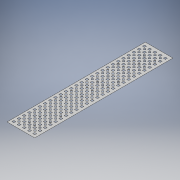
# Autodesk Inventor part: 5sqr metal plate
Saved by Autodesk Inventor 2018 (Build 220112000, 112)
## iProperties
Created: 2018-11-08
Part Number: 5sqr metal plate
Material: Generic
Document SubType Name: Modeling
Designer: USER
Density: 1 g/cm^3
Appearance: Default
Author: USER
Autodesk Inventor part; units mm, degrees
(part 1 of 2)
ref_plane "YZ Plane" through (0, 0, 0) normal (1, 0, 0) x (0, 1, 0)
ref_plane "XZ Plane" through (0, 0, 0) normal (0, 1, 0) x (-1, 0, 0)
ref_plane "XY Plane" through (0, 0, 0) normal (0, 0, 1) x (1, 0, 0)
sketch "Sketch1" plane through (0, 0, 0) normal (0, 1, 0) x (-1, 0, 0)
  line L0 (0, 0) -> (63, 0)
  line L1 (63, 0) -> (63, -315)
  line L2 (63, -315) -> (0, -315)
  line L3 (0, -315) -> (0, 0)
  dimension "d0" = 63
  dimension "d1" = 315
  constraints: 8 end point, 2 parallel, 1 horizontal, 1 perpendicular
  measures "d0" distance of L1.end L2.end
  measures "d1" distance of L0.end L1.end
extrude "Extrusion1" add sketch "Sketch1" along normal blind 0.1
sketch "Sketch2" plane through (0, 0.1, 0) normal (0, 1, 0) x (1, 0, 0)
  line L0 (-58.2087, 6.1745) -> (-53.6367, 6.1745)
  line L1 (-53.6367, 6.1745) -> (-53.6367, 10.7465)
  line L2 (-53.6367, 10.7465) -> (-58.2087, 10.7465)
  line L3 (-58.2087, 10.7465) -> (-58.2087, 6.1745)
  line L4 (-58.2087, 22.6465) -> (-58.2087, 18.0745)
  line L5 (-58.2087, 18.0745) -> (-53.6367, 18.0745)
  line L6 (-53.6367, 18.0745) -> (-53.6367, 22.6465)
  line L7 (-53.6367, 22.6465) -> (-58.2087, 22.6465)
  line L8 (-58.2087, 34.5465) -> (-58.2087, 29.9745)
  line L9 (-58.2087, 29.9745) -> (-53.6367, 29.9745)
  line L10 (-53.6367, 29.9745) -> (-53.6367, 34.5465)
  line L11 (-53.6367, 34.5465) -> (-58.2087, 34.5465)
  line L12 (-58.2087, 46.4465) -> (-58.2087, 41.8745)
  line L13 (-58.2087, 41.8745) -> (-53.6367, 41.8745)
  line L14 (-53.6367, 41.8745) -> (-53.6367, 46.4465)
  line L15 (-53.6367, 46.4465) -> (-58.2087, 46.4465)
  line L16 (-58.2087, 58.3465) -> (-58.2087, 53.7745)
  line L17 (-58.2087, 53.7745) -> (-53.6367, 53.7745)
  line L18 (-53.6367, 53.7745) -> (-53.6367, 58.3465)
  line L19 (-53.6367, 58.3465) -> (-58.2087, 58.3465)
  line L20 (-58.2087, 70.2465) -> (-58.2087, 65.6745)
  line L21 (-58.2087, 65.6745) -> (-53.6367, 65.6745)
  line L22 (-53.6367, 65.6745) -> (-53.6367, 70.2465)
  line L23 (-53.6367, 70.2465) -> (-58.2087, 70.2465)
  line L24 (-58.2087, 82.1465) -> (-58.2087, 77.5745)
  line L25 (-58.2087, 77.5745) -> (-53.6367, 77.5745)
  line L26 (-53.6367, 77.5745) -> (-53.6367, 82.1465)
  line L27 (-53.6367, 82.1465) -> (-58.2087, 82.1465)
  line L28 (-58.2087, 94.0465) -> (-58.2087, 89.4745)
  line L29 (-58.2087, 89.4745) -> (-53.6367, 89.4745)
  line L30 (-53.6367, 89.4745) -> (-53.6367, 94.0465)
  line L31 (-53.6367, 94.0465) -> (-58.2087, 94.0465)
  line L32 (-58.2087, 105.9465) -> (-58.2087, 101.3745)
  line L33 (-58.2087, 101.3745) -> (-53.6367, 101.3745)
  line L34 (-53.6367, 101.3745) -> (-53.6367, 105.9465)
  line L35 (-53.6367, 105.9465) -> (-58.2087, 105.9465)
  line L36 (-58.2087, 117.8465) -> (-58.2087, 113.2745)
  line L37 (-58.2087, 113.2745) -> (-53.6367, 113.2745)
  line L38 (-53.6367, 113.2745) -> (-53.6367, 117.8465)
  line L39 (-53.6367, 117.8465) -> (-58.2087, 117.8465)
  line L40 (-58.2087, 129.7465) -> (-58.2087, 125.1745)
  line L41 (-58.2087, 125.1745) -> (-53.6367, 125.1745)
  line L42 (-53.6367, 125.1745) -> (-53.6367, 129.7465)
  line L43 (-53.6367, 129.7465) -> (-58.2087, 129.7465)
  line L44 (-58.2087, 141.6465) -> (-58.2087, 137.0745)
  line L45 (-58.2087, 137.0745) -> (-53.6367, 137.0745)
  line L46 (-53.6367, 137.0745) -> (-53.6367, 141.6465)
  line L47 (-53.6367, 141.6465) -> (-58.2087, 141.6465)
  line L48 (-58.2087, 153.5465) -> (-58.2087, 148.9745)
  line L49 (-58.2087, 148.9745) -> (-53.6367, 148.9745)
  line L50 (-53.6367, 148.9745) -> (-53.6367, 153.5465)
  line L51 (-53.6367, 153.5465) -> (-58.2087, 153.5465)
  line L52 (-58.2087, 165.4465) -> (-58.2087, 160.8745)
  line L53 (-58.2087, 160.8745) -> (-53.6367, 160.8745)
  line L54 (-53.6367, 160.8745) -> (-53.6367, 165.4465)
  line L55 (-53.6367, 165.4465) -> (-58.2087, 165.4465)
  line L56 (-58.2087, 177.3465) -> (-58.2087, 172.7745)
  line L57 (-58.2087, 172.7745) -> (-53.6367, 172.7745)
  line L58 (-53.6367, 172.7745) -> (-53.6367, 177.3465)
  line L59 (-53.6367, 177.3465) -> (-58.2087, 177.3465)
  line L60 (-58.2087, 189.2465) -> (-58.2087, 184.6745)
  line L61 (-58.2087, 184.6745) -> (-53.6367, 184.6745)
  line L62 (-53.6367, 184.6745) -> (-53.6367, 189.2465)
  line L63 (-53.6367, 189.2465) -> (-58.2087, 189.2465)
  line L64 (-58.2087, 201.1465) -> (-58.2087, 196.5745)
  line L65 (-58.2087, 196.5745) -> (-53.6367, 196.5745)
  line L66 (-53.6367, 196.5745) -> (-53.6367, 201.1465)
  line L67 (-53.6367, 201.1465) -> (-58.2087, 201.1465)
  line L68 (-58.2087, 213.0465) -> (-58.2087, 208.4745)
  line L69 (-58.2087, 208.4745) -> (-53.6367, 208.4745)
  line L70 (-53.6367, 208.4745) -> (-53.6367, 213.0465)
  line L71 (-53.6367, 213.0465) -> (-58.2087, 213.0465)
  line L72 (-58.2087, 224.9465) -> (-58.2087, 220.3745)
  line L73 (-58.2087, 220.3745) -> (-53.6367, 220.3745)
  line L74 (-53.6367, 220.3745) -> (-53.6367, 224.9465)
  line L75 (-53.6367, 224.9465) -> (-58.2087, 224.9465)
  line L76 (-58.2087, 236.8465) -> (-58.2087, 232.2745)
  line L77 (-58.2087, 232.2745) -> (-53.6367, 232.2745)
  line L78 (-53.6367, 232.2745) -> (-53.6367, 236.8465)
  line L79 (-53.6367, 236.8465) -> (-58.2087, 236.8465)
  line L80 (-58.2087, 248.7465) -> (-58.2087, 244.1745)
  line L81 (-58.2087, 244.1745) -> (-53.6367, 244.1745)
  line L82 (-53.6367, 244.1745) -> (-53.6367, 248.7465)
  line L83 (-53.6367, 248.7465) -> (-58.2087, 248.7465)
  line L84 (-58.2087, 260.6465) -> (-58.2087, 256.0745)
  line L85 (-58.2087, 256.0745) -> (-53.6367, 256.0745)
  line L86 (-53.6367, 256.0745) -> (-53.6367, 260.6465)
  line L87 (-53.6367, 260.6465) -> (-58.2087, 260.6465)
  line L88 (-58.2087, 272.5465) -> (-58.2087, 267.9745)
  line L89 (-58.2087, 267.9745) -> (-53.6367, 267.9745)
  line L90 (-53.6367, 267.9745) -> (-53.6367, 272.5465)
  line L91 (-53.6367, 272.5465) -> (-58.2087, 272.5465)
  line L92 (-58.2087, 284.4465) -> (-58.2087, 279.8745)
  line L93 (-58.2087, 279.8745) -> (-53.6367, 279.8745)
  line L94 (-53.6367, 279.8745) -> (-53.6367, 284.4465)
  line L95 (-53.6367, 284.4465) -> (-58.2087, 284.4465)
  line L96 (-58.2087, 296.3465) -> (-58.2087, 291.7745)
  line L97 (-58.2087, 291.7745) -> (-53.6367, 291.7745)
  line L98 (-53.6367, 291.7745) -> (-53.6367, 296.3465)
  line L99 (-53.6367, 296.3465) -> (-58.2087, 296.3465)
  line L100 (-58.2087, 308.2465) -> (-58.2087, 303.6745)
  line L101 (-58.2087, 303.6745) -> (-53.6367, 303.6745)
  line L102 (-53.6367, 303.6745) -> (-53.6367, 308.2465)
  line L103 (-53.6367, 308.2465) -> (-58.2087, 308.2465)
  line L104 (-46.3087, 10.7465) -> (-46.3087, 6.1745)
  line L105 (-46.3087, 6.1745) -> (-41.7367, 6.1745)
  line L106 (-41.7367, 6.1745) -> (-41.7367, 10.7465)
  line L107 (-41.7367, 10.7465) -> (-46.3087, 10.7465)
  line L108 (-46.3087, 22.6465) -> (-46.3087, 18.0745)
  line L109 (-46.3087, 18.0745) -> (-41.7367, 18.0745)
  line L110 (-41.7367, 18.0745) -> (-41.7367, 22.6465)
  line L111 (-41.7367, 22.6465) -> (-46.3087, 22.6465)
  line L112 (-46.3087, 34.5465) -> (-46.3087, 29.9745)
  line L113 (-46.3087, 29.9745) -> (-41.7367, 29.9745)
  line L114 (-41.7367, 29.9745) -> (-41.7367, 34.5465)
  line L115 (-41.7367, 34.5465) -> (-46.3087, 34.5465)
  line L116 (-46.3087, 46.4465) -> (-46.3087, 41.8745)
  line L117 (-46.3087, 41.8745) -> (-41.7367, 41.8745)
  line L118 (-41.7367, 41.8745) -> (-41.7367, 46.4465)
  line L119 (-41.7367, 46.4465) -> (-46.3087, 46.4465)
  line L120 (-46.3087, 58.3465) -> (-46.3087, 53.7745)
  line L121 (-46.3087, 53.7745) -> (-41.7367, 53.7745)
  line L122 (-41.7367, 53.7745) -> (-41.7367, 58.3465)
  line L123 (-41.7367, 58.3465) -> (-46.3087, 58.3465)
  line L124 (-46.3087, 70.2465) -> (-46.3087, 65.6745)
  line L125 (-46.3087, 65.6745) -> (-41.7367, 65.6745)
  line L126 (-41.7367, 65.6745) -> (-41.7367, 70.2465)
  line L127 (-41.7367, 70.2465) -> (-46.3087, 70.2465)
  line L128 (-46.3087, 82.1465) -> (-46.3087, 77.5745)
  line L129 (-46.3087, 77.5745) -> (-41.7367, 77.5745)
  line L130 (-41.7367, 77.5745) -> (-41.7367, 82.1465)
  line L131 (-41.7367, 82.1465) -> (-46.3087, 82.1465)
  line L132 (-46.3087, 94.0465) -> (-46.3087, 89.4745)
  line L133 (-46.3087, 89.4745) -> (-41.7367, 89.4745)
  line L134 (-41.7367, 89.4745) -> (-41.7367, 94.0465)
  line L135 (-41.7367, 94.0465) -> (-46.3087, 94.0465)
  line L136 (-46.3087, 105.9465) -> (-46.3087, 101.3745)
  line L137 (-46.3087, 101.3745) -> (-41.7367, 101.3745)
  line L138 (-41.7367, 101.3745) -> (-41.7367, 105.9465)
  line L139 (-41.7367, 105.9465) -> (-46.3087, 105.9465)
  line L140 (-46.3087, 117.8465) -> (-46.3087, 113.2745)
  line L141 (-46.3087, 113.2745) -> (-41.7367, 113.2745)
  line L142 (-41.7367, 113.2745) -> (-41.7367, 117.8465)
  line L143 (-41.7367, 117.8465) -> (-46.3087, 117.8465)
  line L144 (-46.3087, 129.7465) -> (-46.3087, 125.1745)
  line L145 (-46.3087, 125.1745) -> (-41.7367, 125.1745)
  line L146 (-41.7367, 125.1745) -> (-41.7367, 129.7465)
  line L147 (-41.7367, 129.7465) -> (-46.3087, 129.7465)
  line L148 (-46.3087, 141.6465) -> (-46.3087, 137.0745)
  line L149 (-46.3087, 137.0745) -> (-41.7367, 137.0745)
  line L150 (-41.7367, 137.0745) -> (-41.7367, 141.6465)
  line L151 (-41.7367, 141.6465) -> (-46.3087, 141.6465)
  line L152 (-46.3087, 153.5465) -> (-46.3087, 148.9745)
  line L153 (-46.3087, 148.9745) -> (-41.7367, 148.9745)
  line L154 (-41.7367, 148.9745) -> (-41.7367, 153.5465)
  line L155 (-41.7367, 153.5465) -> (-46.3087, 153.5465)
  line L156 (-46.3087, 165.4465) -> (-46.3087, 160.8745)
  line L157 (-46.3087, 160.8745) -> (-41.7367, 160.8745)
  line L158 (-41.7367, 160.8745) -> (-41.7367, 165.4465)
  line L159 (-41.7367, 165.4465) -> (-46.3087, 165.4465)
  line L160 (-46.3087, 177.3465) -> (-46.3087, 172.7745)
  line L161 (-46.3087, 172.7745) -> (-41.7367, 172.7745)
  line L162 (-41.7367, 172.7745) -> (-41.7367, 177.3465)
  line L163 (-41.7367, 177.3465) -> (-46.3087, 177.3465)
  line L164 (-46.3087, 189.2465) -> (-46.3087, 184.6745)
  line L165 (-46.3087, 184.6745) -> (-41.7367, 184.6745)
  line L166 (-41.7367, 184.6745) -> (-41.7367, 189.2465)
  line L167 (-41.7367, 189.2465) -> (-46.3087, 189.2465)
  line L168 (-46.3087, 201.1465) -> (-46.3087, 196.5745)
  line L169 (-46.3087, 196.5745) -> (-41.7367, 196.5745)
  line L170 (-41.7367, 196.5745) -> (-41.7367, 201.1465)
  line L171 (-41.7367, 201.1465) -> (-46.3087, 201.1465)
  line L172 (-46.3087, 213.0465) -> (-46.3087, 208.4745)
  line L173 (-46.3087, 208.4745) -> (-41.7367, 208.4745)
  line L174 (-41.7367, 208.4745) -> (-41.7367, 213.0465)
  line L175 (-41.7367, 213.0465) -> (-46.3087, 213.0465)
  line L176 (-46.3087, 224.9465) -> (-46.3087, 220.3745)
  line L177 (-46.3087, 220.3745) -> (-41.7367, 220.3745)
  line L178 (-41.7367, 220.3745) -> (-41.7367, 224.9465)
  line L179 (-41.7367, 224.9465) -> (-46.3087, 224.9465)
  line L180 (-46.3087, 236.8465) -> (-46.3087, 232.2745)
  line L181 (-46.3087, 232.2745) -> (-41.7367, 232.2745)
  line L182 (-41.7367, 232.2745) -> (-41.7367, 236.8465)
  line L183 (-41.7367, 236.8465) -> (-46.3087, 236.8465)
  line L184 (-46.3087, 248.7465) -> (-46.3087, 244.1745)
  line L185 (-46.3087, 244.1745) -> (-41.7367, 244.1745)
  line L186 (-41.7367, 244.1745) -> (-41.7367, 248.7465)
  line L187 (-41.7367, 248.7465) -> (-46.3087, 248.7465)
  line L188 (-46.3087, 260.6465) -> (-46.3087, 256.0745)
  line L189 (-46.3087, 256.0745) -> (-41.7367, 256.0745)
  line L190 (-41.7367, 256.0745) -> (-41.7367, 260.6465)
  line L191 (-41.7367, 260.6465) -> (-46.3087, 260.6465)
  line L192 (-46.3087, 272.5465) -> (-46.3087, 267.9745)
  line L193 (-46.3087, 267.9745) -> (-41.7367, 267.9745)
  line L194 (-41.7367, 267.9745) -> (-41.7367, 272.5465)
  line L195 (-41.7367, 272.5465) -> (-46.3087, 272.5465)
  line L196 (-46.3087, 284.4465) -> (-46.3087, 279.8745)
  line L197 (-46.3087, 279.8745) -> (-41.7367, 279.8745)
  line L198 (-41.7367, 279.8745) -> (-41.7367, 284.4465)
  line L199 (-41.7367, 284.4465) -> (-46.3087, 284.4465)
  line L200 (-46.3087, 296.3465) -> (-46.3087, 291.7745)
  line L201 (-46.3087, 291.7745) -> (-41.7367, 291.7745)
  line L202 (-41.7367, 291.7745) -> (-41.7367, 296.3465)
  line L203 (-41.7367, 296.3465) -> (-46.3087, 296.3465)
  line L204 (-46.3087, 308.2465) -> (-46.3087, 303.6745)
  line L205 (-46.3087, 303.6745) -> (-41.7367, 303.6745)
  line L206 (-41.7367, 303.6745) -> (-41.7367, 308.2465)
  line L207 (-41.7367, 308.2465) -> (-46.3087, 308.2465)
  line L208 (-34.4087, 10.7465) -> (-34.4087, 6.1745)
  line L209 (-34.4087, 6.1745) -> (-29.8367, 6.1745)
  line L210 (-29.8367, 6.1745) -> (-29.8367, 10.7465)
  line L211 (-29.8367, 10.7465) -> (-34.4087, 10.7465)
  line L212 (-34.4087, 22.6465) -> (-34.4087, 18.0745)
  line L213 (-34.4087, 18.0745) -> (-29.8367, 18.0745)
  line L214 (-29.8367, 18.0745) -> (-29.8367, 22.6465)
  line L215 (-29.8367, 22.6465) -> (-34.4087, 22.6465)
  line L216 (-34.4087, 34.5465) -> (-34.4087, 29.9745)
  line L217 (-34.4087, 29.9745) -> (-29.8367, 29.9745)
  line L218 (-29.8367, 29.9745) -> (-29.8367, 34.5465)
  line L219 (-29.8367, 34.5465) -> (-34.4087, 34.5465)
  line L220 (-34.4087, 46.4465) -> (-34.4087, 41.8745)
  line L221 (-34.4087, 41.8745) -> (-29.8367, 41.8745)
  line L222 (-29.8367, 41.8745) -> (-29.8367, 46.4465)
  line L223 (-29.8367, 46.4465) -> (-34.4087, 46.4465)
  line L224 (-34.4087, 58.3465) -> (-34.4087, 53.7745)
  line L225 (-34.4087, 53.7745) -> (-29.8367, 53.7745)
  line L226 (-29.8367, 53.7745) -> (-29.8367, 58.3465)
  line L227 (-29.8367, 58.3465) -> (-34.4087, 58.3465)
  line L228 (-34.4087, 70.2465) -> (-34.4087, 65.6745)
  line L229 (-34.4087, 65.6745) -> (-29.8367, 65.6745)
  line L230 (-29.8367, 65.6745) -> (-29.8367, 70.2465)
  line L231 (-29.8367, 70.2465) -> (-34.4087, 70.2465)
  line L232 (-34.4087, 82.1465) -> (-34.4087, 77.5745)
  line L233 (-34.4087, 77.5745) -> (-29.8367, 77.5745)
  line L234 (-29.8367, 77.5745) -> (-29.8367, 82.1465)
  line L235 (-29.8367, 82.1465) -> (-34.4087, 82.1465)
  line L236 (-34.4087, 94.0465) -> (-34.4087, 89.4745)
  line L237 (-34.4087, 89.4745) -> (-29.8367, 89.4745)
  line L238 (-29.8367, 89.4745) -> (-29.8367, 94.0465)
  line L239 (-29.8367, 94.0465) -> (-34.4087, 94.0465)
  line L240 (-34.4087, 105.9465) -> (-34.4087, 101.3745)
  line L241 (-34.4087, 101.3745) -> (-29.8367, 101.3745)
  line L242 (-29.8367, 101.3745) -> (-29.8367, 105.9465)
  line L243 (-29.8367, 105.9465) -> (-34.4087, 105.9465)
  line L244 (-34.4087, 117.8465) -> (-34.4087, 113.2745)
  line L245 (-34.4087, 113.2745) -> (-29.8367, 113.2745)
  line L246 (-29.8367, 113.2745) -> (-29.8367, 117.8465)
  line L247 (-29.8367, 117.8465) -> (-34.4087, 117.8465)
  line L248 (-34.4087, 129.7465) -> (-34.4087, 125.1745)
  line L249 (-34.4087, 125.1745) -> (-29.8367, 125.1745)
  line L250 (-29.8367, 125.1745) -> (-29.8367, 129.7465)
  line L251 (-29.8367, 129.7465) -> (-34.4087, 129.7465)
  line L252 (-34.4087, 141.6465) -> (-34.4087, 137.0745)
  line L253 (-34.4087, 137.0745) -> (-29.8367, 137.0745)
  line L254 (-29.8367, 137.0745) -> (-29.8367, 141.6465)
  line L255 (-29.8367, 141.6465) -> (-34.4087, 141.6465)
  line L256 (-34.4087, 153.5465) -> (-34.4087, 148.9745)
  line L257 (-34.4087, 148.9745) -> (-29.8367, 148.9745)
  line L258 (-29.8367, 148.9745) -> (-29.8367, 153.5465)
  line L259 (-29.8367, 153.5465) -> (-34.4087, 153.5465)
  line L260 (-34.4087, 165.4465) -> (-34.4087, 160.8745)
  line L261 (-34.4087, 160.8745) -> (-29.8367, 160.8745)
  line L262 (-29.8367, 160.8745) -> (-29.8367, 165.4465)
  line L263 (-29.8367, 165.4465) -> (-34.4087, 165.4465)
  line L264 (-34.4087, 177.3465) -> (-34.4087, 172.7745)
  line L265 (-34.4087, 172.7745) -> (-29.8367, 172.7745)
  line L266 (-29.8367, 172.7745) -> (-29.8367, 177.3465)
  line L267 (-29.8367, 177.3465) -> (-34.4087, 177.3465)
  line L268 (-34.4087, 189.2465) -> (-34.4087, 184.6745)
  line L269 (-34.4087, 184.6745) -> (-29.8367, 184.6745)
  line L270 (-29.8367, 184.6745) -> (-29.8367, 189.2465)
  line L271 (-29.8367, 189.2465) -> (-34.4087, 189.2465)
  line L272 (-34.4087, 201.1465) -> (-34.4087, 196.5745)
  line L273 (-34.4087, 196.5745) -> (-29.8367, 196.5745)
  line L274 (-29.8367, 196.5745) -> (-29.8367, 201.1465)
  line L275 (-29.8367, 201.1465) -> (-34.4087, 201.1465)
  line L276 (-34.4087, 213.0465) -> (-34.4087, 208.4745)
  line L277 (-34.4087, 208.4745) -> (-29.8367, 208.4745)
  line L278 (-29.8367, 208.4745) -> (-29.8367, 213.0465)
  line L279 (-29.8367, 213.0465) -> (-34.4087, 213.0465)
  line L280 (-34.4087, 224.9465) -> (-34.4087, 220.3745)
  line L281 (-34.4087, 220.3745) -> (-29.8367, 220.3745)
  line L282 (-29.8367, 220.3745) -> (-29.8367, 224.9465)
  line L283 (-29.8367, 224.9465) -> (-34.4087, 224.9465)
  line L284 (-34.4087, 236.8465) -> (-34.4087, 232.2745)
  line L285 (-34.4087, 232.2745) -> (-29.8367, 232.2745)
  line L286 (-29.8367, 232.2745) -> (-29.8367, 236.8465)
  line L287 (-29.8367, 236.8465) -> (-34.4087, 236.8465)
  line L288 (-34.4087, 248.7465) -> (-34.4087, 244.1745)
  line L289 (-34.4087, 244.1745) -> (-29.8367, 244.1745)
  line L290 (-29.8367, 244.1745) -> (-29.8367, 248.7465)
  line L291 (-29.8367, 248.7465) -> (-34.4087, 248.7465)
  line L292 (-34.4087, 260.6465) -> (-34.4087, 256.0745)
  line L293 (-34.4087, 256.0745) -> (-29.8367, 256.0745)
  line L294 (-29.8367, 256.0745) -> (-29.8367, 260.6465)
  line L295 (-29.8367, 260.6465) -> (-34.4087, 260.6465)
  line L296 (-34.4087, 272.5465) -> (-34.4087, 267.9745)
  line L297 (-34.4087, 267.9745) -> (-29.8367, 267.9745)
  line L298 (-29.8367, 267.9745) -> (-29.8367, 272.5465)
  line L299 (-29.8367, 272.5465) -> (-34.4087, 272.5465)
  line L300 (-34.4087, 284.4465) -> (-34.4087, 279.8745)
  line L301 (-34.4087, 279.8745) -> (-29.8367, 279.8745)
  line L302 (-29.8367, 279.8745) -> (-29.8367, 284.4465)
  line L303 (-29.8367, 284.4465) -> (-34.4087, 284.4465)
  line L304 (-34.4087, 296.3465) -> (-34.4087, 291.7745)
  line L305 (-34.4087, 291.7745) -> (-29.8367, 291.7745)
  line L306 (-29.8367, 291.7745) -> (-29.8367, 296.3465)
  line L307 (-29.8367, 296.3465) -> (-34.4087, 296.3465)
  line L308 (-34.4087, 308.2465) -> (-34.4087, 303.6745)
  line L309 (-34.4087, 303.6745) -> (-29.8367, 303.6745)
  line L310 (-29.8367, 303.6745) -> (-29.8367, 308.2465)
  line L311 (-29.8367, 308.2465) -> (-34.4087, 308.2465)
  line L312 (-22.5087, 10.7465) -> (-22.5087, 6.1745)
  line L313 (-22.5087, 6.1745) -> (-17.9367, 6.1745)
  line L314 (-17.9367, 6.1745) -> (-17.9367, 10.7465)
  line L315 (-17.9367, 10.7465) -> (-22.5087, 10.7465)
  line L316 (-22.5087, 22.6465) -> (-22.5087, 18.0745)
  line L317 (-22.5087, 18.0745) -> (-17.9367, 18.0745)
  line L318 (-17.9367, 18.0745) -> (-17.9367, 22.6465)
  line L319 (-17.9367, 22.6465) -> (-22.5087, 22.6465)
  line L320 (-22.5087, 34.5465) -> (-22.5087, 29.9745)
  line L321 (-22.5087, 29.9745) -> (-17.9367, 29.9745)
  line L322 (-17.9367, 29.9745) -> (-17.9367, 34.5465)
  line L323 (-17.9367, 34.5465) -> (-22.5087, 34.5465)
  line L324 (-22.5087, 46.4465) -> (-22.5087, 41.8745)
  line L325 (-22.5087, 41.8745) -> (-17.9367, 41.8745)
  line L326 (-17.9367, 41.8745) -> (-17.9367, 46.4465)
  line L327 (-17.9367, 46.4465) -> (-22.5087, 46.4465)
  line L328 (-22.5087, 58.3465) -> (-22.5087, 53.7745)
  line L329 (-22.5087, 53.7745) -> (-17.9367, 53.7745)
  line L330 (-17.9367, 53.7745) -> (-17.9367, 58.3465)
  line L331 (-17.9367, 58.3465) -> (-22.5087, 58.3465)
  line L332 (-22.5087, 70.2465) -> (-22.5087, 65.6745)
  line L333 (-22.5087, 65.6745) -> (-17.9367, 65.6745)
  line L334 (-17.9367, 65.6745) -> (-17.9367, 70.2465)
  line L335 (-17.9367, 70.2465) -> (-22.5087, 70.2465)
  line L336 (-22.5087, 82.1465) -> (-22.5087, 77.5745)
  line L337 (-22.5087, 77.5745) -> (-17.9367, 77.5745)
  line L338 (-17.9367, 77.5745) -> (-17.9367, 82.1465)
  line L339 (-17.9367, 82.1465) -> (-22.5087, 82.1465)
  line L340 (-22.5087, 94.0465) -> (-22.5087, 89.4745)
  line L341 (-22.5087, 89.4745) -> (-17.9367, 89.4745)
  line L342 (-17.9367, 89.4745) -> (-17.9367, 94.0465)
  line L343 (-17.9367, 94.0465) -> (-22.5087, 94.0465)
  line L344 (-22.5087, 105.9465) -> (-22.5087, 101.3745)
  line L345 (-22.5087, 101.3745) -> (-17.9367, 101.3745)
  line L346 (-17.9367, 101.3745) -> (-17.9367, 105.9465)
  line L347 (-17.9367, 105.9465) -> (-22.5087, 105.9465)
  line L348 (-22.5087, 117.8465) -> (-22.5087, 113.2745)
  line L349 (-22.5087, 113.2745) -> (-17.9367, 113.2745)
  line L350 (-17.9367, 113.2745) -> (-17.9367, 117.8465)
  line L351 (-17.9367, 117.8465) -> (-22.5087, 117.8465)
  line L352 (-22.5087, 129.7465) -> (-22.5087, 125.1745)
  line L353 (-22.5087, 125.1745) -> (-17.9367, 125.1745)
  line L354 (-17.9367, 125.1745) -> (-17.9367, 129.7465)
  line L355 (-17.9367, 129.7465) -> (-22.5087, 129.7465)
  line L356 (-22.5087, 141.6465) -> (-22.5087, 137.0745)
  line L357 (-22.5087, 137.0745) -> (-17.9367, 137.0745)
  line L358 (-17.9367, 137.0745) -> (-17.9367, 141.6465)
  line L359 (-17.9367, 141.6465) -> (-22.5087, 141.6465)
  line L360 (-22.5087, 153.5465) -> (-22.5087, 148.9745)
  line L361 (-22.5087, 148.9745) -> (-17.9367, 148.9745)
  line L362 (-17.9367, 148.9745) -> (-17.9367, 153.5465)
  line L363 (-17.9367, 153.5465) -> (-22.5087, 153.5465)
  line L364 (-22.5087, 165.4465) -> (-22.5087, 160.8745)
  line L365 (-22.5087, 160.8745) -> (-17.9367, 160.8745)
  line L366 (-17.9367, 160.8745) -> (-17.9367, 165.4465)
  line L367 (-17.9367, 165.4465) -> (-22.5087, 165.4465)
  line L368 (-22.5087, 177.3465) -> (-22.5087, 172.7745)
  line L369 (-22.5087, 172.7745) -> (-17.9367, 172.7745)
  line L370 (-17.9367, 172.7745) -> (-17.9367, 177.3465)
  line L371 (-17.9367, 177.3465) -> (-22.5087, 177.3465)
  line L372 (-22.5087, 189.2465) -> (-22.5087, 184.6745)
  line L373 (-22.5087, 184.6745) -> (-17.9367, 184.6745)
  line L374 (-17.9367, 184.6745) -> (-17.9367, 189.2465)
  line L375 (-17.9367, 189.2465) -> (-22.5087, 189.2465)
  line L376 (-22.5087, 201.1465) -> (-22.5087, 196.5745)
  line L377 (-22.5087, 196.5745) -> (-17.9367, 196.5745)
  line L378 (-17.9367, 196.5745) -> (-17.9367, 201.1465)
  line L379 (-17.9367, 201.1465) -> (-22.5087, 201.1465)
  line L380 (-22.5087, 213.0465) -> (-22.5087, 208.4745)
  line L381 (-22.5087, 208.4745) -> (-17.9367, 208.4745)
  line L382 (-17.9367, 208.4745) -> (-17.9367, 213.0465)
  line L383 (-17.9367, 213.0465) -> (-22.5087, 213.0465)
  line L384 (-22.5087, 224.9465) -> (-22.5087, 220.3745)
  line L385 (-22.5087, 220.3745) -> (-17.9367, 220.3745)
  line L386 (-17.9367, 220.3745) -> (-17.9367, 224.9465)
  line L387 (-17.9367, 224.9465) -> (-22.5087, 224.9465)
  line L388 (-22.5087, 236.8465) -> (-22.5087, 232.2745)
  line L389 (-22.5087, 232.2745) -> (-17.9367, 232.2745)
  line L390 (-17.9367, 232.2745) -> (-17.9367, 236.8465)
  line L391 (-17.9367, 236.8465) -> (-22.5087, 236.8465)
  line L392 (-22.5087, 248.7465) -> (-22.5087, 244.1745)
  line L393 (-22.5087, 244.1745) -> (-17.9367, 244.1745)
  line L394 (-17.9367, 244.1745) -> (-17.9367, 248.7465)
  line L395 (-17.9367, 248.7465) -> (-22.5087, 248.7465)
  line L396 (-22.5087, 260.6465) -> (-22.5087, 256.0745)
  line L397 (-22.5087, 256.0745) -> (-17.9367, 256.0745)
  line L398 (-17.9367, 256.0745) -> (-17.9367, 260.6465)
  line L399 (-17.9367, 260.6465) -> (-22.5087, 260.6465)
  line L400 (-22.5087, 272.5465) -> (-22.5087, 267.9745)
  line L401 (-22.5087, 267.9745) -> (-17.9367, 267.9745)
  line L402 (-17.9367, 267.9745) -> (-17.9367, 272.5465)
  line L403 (-17.9367, 272.5465) -> (-22.5087, 272.5465)
  line L404 (-22.5087, 284.4465) -> (-22.5087, 279.8745)
  line L405 (-22.5087, 279.8745) -> (-17.9367, 279.8745)
  line L406 (-17.9367, 279.8745) -> (-17.9367, 284.4465)
  line L407 (-17.9367, 284.4465) -> (-22.5087, 284.4465)
  line L408 (-22.5087, 296.3465) -> (-22.5087, 291.7745)
  line L409 (-22.5087, 291.7745) -> (-17.9367, 291.7745)
  line L410 (-17.9367, 291.7745) -> (-17.9367, 296.3465)
  line L411 (-17.9367, 296.3465) -> (-22.5087, 296.3465)
  line L412 (-22.5087, 308.2465) -> (-22.5087, 303.6745)
  line L413 (-22.5087, 303.6745) -> (-17.9367, 303.6745)
  line L414 (-17.9367, 303.6745) -> (-17.9367, 308.2465)
  line L415 (-17.9367, 308.2465) -> (-22.5087, 308.2465)
  line L416 (-10.6087, 10.7465) -> (-10.6087, 6.1745)
  line L417 (-10.6087, 6.1745) -> (-6.0367, 6.1745)
  line L418 (-6.0367, 6.1745) -> (-6.0367, 10.7465)
  line L419 (-6.0367, 10.7465) -> (-10.6087, 10.7465)
  line L420 (-10.6087, 22.6465) -> (-10.6087, 18.0745)
  line L421 (-10.6087, 18.0745) -> (-6.0367, 18.0745)
  line L422 (-6.0367, 18.0745) -> (-6.0367, 22.6465)
  line L423 (-6.0367, 22.6465) -> (-10.6087, 22.6465)
  line L424 (-10.6087, 34.5465) -> (-10.6087, 29.9745)
  line L425 (-10.6087, 29.9745) -> (-6.0367, 29.9745)
  line L426 (-6.0367, 29.9745) -> (-6.0367, 34.5465)
  line L427 (-6.0367, 34.5465) -> (-10.6087, 34.5465)
  line L428 (-10.6087, 46.4465) -> (-10.6087, 41.8745)
  line L429 (-10.6087, 41.8745) -> (-6.0367, 41.8745)
  line L430 (-6.0367, 41.8745) -> (-6.0367, 46.4465)
  line L431 (-6.0367, 46.4465) -> (-10.6087, 46.4465)
  line L432 (-10.6087, 58.3465) -> (-10.6087, 53.7745)
  line L433 (-10.6087, 53.7745) -> (-6.0367, 53.7745)
  line L434 (-6.0367, 53.7745) -> (-6.0367, 58.3465)
  line L435 (-6.0367, 58.3465) -> (-10.6087, 58.3465)
  line L436 (-10.6087, 70.2465) -> (-10.6087, 65.6745)
  line L437 (-10.6087, 65.6745) -> (-6.0367, 65.6745)
  line L438 (-6.0367, 65.6745) -> (-6.0367, 70.2465)
  line L439 (-6.0367, 70.2465) -> (-10.6087, 70.2465)
  line L440 (-10.6087, 82.1465) -> (-10.6087, 77.5745)
  line L441 (-10.6087, 77.5745) -> (-6.0367, 77.5745)
  line L442 (-6.0367, 77.5745) -> (-6.0367, 82.1465)
  line L443 (-6.0367, 82.1465) -> (-10.6087, 82.1465)
  line L444 (-10.6087, 94.0465) -> (-10.6087, 89.4745)
  line L445 (-10.6087, 89.4745) -> (-6.0367, 89.4745)
  line L446 (-6.0367, 89.4745) -> (-6.0367, 94.0465)
  line L447 (-6.0367, 94.0465) -> (-10.6087, 94.0465)
  line L448 (-10.6087, 105.9465) -> (-10.6087, 101.3745)
  line L449 (-10.6087, 101.3745) -> (-6.0367, 101.3745)
  line L450 (-6.0367, 101.3745) -> (-6.0367, 105.9465)
  line L451 (-6.0367, 105.9465) -> (-10.6087, 105.9465)
  line L452 (-10.6087, 117.8465) -> (-10.6087, 113.2745)
  line L453 (-10.6087, 113.2745) -> (-6.0367, 113.2745)
  line L454 (-6.0367, 113.2745) -> (-6.0367, 117.8465)
  line L455 (-6.0367, 117.8465) -> (-10.6087, 117.8465)
  line L456 (-10.6087, 129.7465) -> (-10.6087, 125.1745)
  line L457 (-10.6087, 125.1745) -> (-6.0367, 125.1745)
  line L458 (-6.0367, 125.1745) -> (-6.0367, 129.7465)
  line L459 (-6.0367, 129.7465) -> (-10.6087, 129.7465)
  line L460 (-10.6087, 141.6465) -> (-10.6087, 137.0745)
  line L461 (-10.6087, 137.0745) -> (-6.0367, 137.0745)
  line L462 (-6.0367, 137.0745) -> (-6.0367, 141.6465)
  line L463 (-6.0367, 141.6465) -> (-10.6087, 141.6465)
  line L464 (-10.6087, 153.5465) -> (-10.6087, 148.9745)
  line L465 (-10.6087, 148.9745) -> (-6.0367, 148.9745)
  line L466 (-6.0367, 148.9745) -> (-6.0367, 153.5465)
  line L467 (-6.0367, 153.5465) -> (-10.6087, 153.5465)
  line L468 (-10.6087, 165.4465) -> (-10.6087, 160.8745)
  line L469 (-10.6087, 160.8745) -> (-6.0367, 160.8745)
  line L470 (-6.0367, 160.8745) -> (-6.0367, 165.4465)
  line L471 (-6.0367, 165.4465) -> (-10.6087, 165.4465)
  line L472 (-10.6087, 177.3465) -> (-10.6087, 172.7745)
  line L473 (-10.6087, 172.7745) -> (-6.0367, 172.7745)
  line L474 (-6.0367, 172.7745) -> (-6.0367, 177.3465)
  line L475 (-6.0367, 177.3465) -> (-10.6087, 177.3465)
  line L476 (-10.6087, 189.2465) -> (-10.6087, 184.6745)
  line L477 (-10.6087, 184.6745) -> (-6.0367, 184.6745)
  line L478 (-6.0367, 184.6745) -> (-6.0367, 189.2465)
  line L479 (-6.0367, 189.2465) -> (-10.6087, 189.2465)
  line L480 (-10.6087, 201.1465) -> (-10.6087, 196.5745)
  line L481 (-10.6087, 196.5745) -> (-6.0367, 196.5745)
  line L482 (-6.0367, 196.5745) -> (-6.0367, 201.1465)
  line L483 (-6.0367, 201.1465) -> (-10.6087, 201.1465)
  line L484 (-10.6087, 213.0465) -> (-10.6087, 208.4745)
  line L485 (-10.6087, 208.4745) -> (-6.0367, 208.4745)
  line L486 (-6.0367, 208.4745) -> (-6.0367, 213.0465)
  line L487 (-6.0367, 213.0465) -> (-10.6087, 213.0465)
  line L488 (-10.6087, 224.9465) -> (-10.6087, 220.3745)
  line L489 (-10.6087, 220.3745) -> (-6.0367, 220.3745)
  line L490 (-6.0367, 220.3745) -> (-6.0367, 224.9465)
  line L491 (-6.0367, 224.9465) -> (-10.6087, 224.9465)
  line L492 (-10.6087, 236.8465) -> (-10.6087, 232.2745)
  line L493 (-10.6087, 232.2745) -> (-6.0367, 232.2745)
  line L494 (-6.0367, 232.2745) -> (-6.0367, 236.8465)
  line L495 (-6.0367, 236.8465) -> (-10.6087, 236.8465)
  line L496 (-10.6087, 248.7465) -> (-10.6087, 244.1745)
  line L497 (-10.6087, 244.1745) -> (-6.0367, 244.1745)
  line L498 (-6.0367, 244.1745) -> (-6.0367, 248.7465)
  line L499 (-6.0367, 248.7465) -> (-10.6087, 248.7465)
  line L500 (-10.6087, 260.6465) -> (-10.6087, 256.0745)
  line L501 (-10.6087, 256.0745) -> (-6.0367, 256.0745)
  line L502 (-6.0367, 256.0745) -> (-6.0367, 260.6465)
  line L503 (-6.0367, 260.6465) -> (-10.6087, 260.6465)
  line L504 (-10.6087, 272.5465) -> (-10.6087, 267.9745)
  line L505 (-10.6087, 267.9745) -> (-6.0367, 267.9745)
  line L506 (-6.0367, 267.9745) -> (-6.0367, 272.5465)
  line L507 (-6.0367, 272.5465) -> (-10.6087, 272.5465)
  line L508 (-10.6087, 284.4465) -> (-10.6087, 279.8745)
  line L509 (-10.6087, 279.8745) -> (-6.0367, 279.8745)
  line L510 (-6.0367, 279.8745) -> (-6.0367, 284.4465)
  line L511 (-6.0367, 284.4465) -> (-10.6087, 284.4465)
  line L512 (-10.6087, 296.3465) -> (-10.6087, 291.7745)
  line L513 (-10.6087, 291.7745) -> (-6.0367, 291.7745)
  line L514 (-6.0367, 291.7745) -> (-6.0367, 296.3465)
  line L515 (-6.0367, 296.3465) -> (-10.6087, 296.3465)
  line L516 (-10.6087, 308.2465) -> (-10.6087, 303.6745)
  line L517 (-10.6087, 303.6745) -> (-6.0367, 303.6745)
  line L518 (-6.0367, 303.6745) -> (-6.0367, 308.2465)
  line L519 (-6.0367, 308.2465) -> (-10.6087, 308.2465)
  line L520 (-50.0217, 11.9442) -> (-52.7477, 14.6702)
  line L521 (-52.7477, 14.6702) -> (-50.0748, 17.3431)
  line L522 (-50.0748, 17.3431) -> (-47.3488, 14.6171)
  line L523 (-47.3488, 14.6171) -> (-50.0217, 11.9442)
  line L524 (-50.0217, 11.9442) -> (-50.0748, 17.3431) construction
  line L525 (-52.7477, 14.6702) -> (-47.3488, 14.6171) construction
  line L526 (-38.0237, 11.9442) -> (-35.2976, 14.6702)
  line L527 (-35.2976, 14.6702) -> (-37.9706, 17.3431)
  line L528 (-37.9706, 17.3431) -> (-40.6966, 14.6171)
  line L529 (-40.6966, 14.6171) -> (-38.0237, 11.9442)
  line L530 (-14.2237, 11.9442) -> (-11.4976, 14.6702)
  line L531 (-11.4976, 14.6702) -> (-14.1706, 17.3431)
  line L532 (-14.1706, 17.3431) -> (-16.8966, 14.6171)
  line L533 (-16.8966, 14.6171) -> (-14.2237, 11.9442)
  line L534 (-26.2217, 11.9442) -> (-28.9477, 14.6702)
  line L535 (-28.9477, 14.6702) -> (-26.2748, 17.3431)
  line L536 (-26.2748, 17.3431) -> (-23.5488, 14.6171)
  line L537 (-23.5488, 14.6171) -> (-26.2217, 11.9442)
  line L538 (-50.0217, 28.7769) -> (-52.7477, 26.0508)
  line L539 (-52.7477, 26.0508) -> (-50.0748, 23.3779)
  line L540 (-50.0748, 23.3779) -> (-47.3488, 26.1039)
  line L541 (-47.3488, 26.1039) -> (-50.0217, 28.7769)
  line L542 (-50.0217, 28.7769) -> (-50.0748, 23.3779) construction
  line L543 (-52.7477, 26.0508) -> (-47.3488, 26.1039) construction
  line L544 (-38.0237, 28.7769) -> (-35.2976, 26.0508)
  line L545 (-35.2976, 26.0508) -> (-37.9706, 23.3779)
  line L546 (-37.9706, 23.3779) -> (-40.6966, 26.1039)
  line L547 (-40.6966, 26.1039) -> (-38.0237, 28.7769)
  line L548 (-14.2237, 28.7769) -> (-11.4976, 26.0508)
  line L549 (-11.4976, 26.0508) -> (-14.1706, 23.3779)
  line L550 (-14.1706, 23.3779) -> (-16.8966, 26.1039)
  line L551 (-16.8966, 26.1039) -> (-14.2237, 28.7769)
  line L552 (-23.5488, 26.1039) -> (-26.2217, 28.7769)
  line L553 (-26.2748, 23.3779) -> (-23.5488, 26.1039)
  line L554 (-28.9477, 26.0508) -> (-26.2748, 23.3779)
  line L555 (-26.2217, 28.7769) -> (-28.9477, 26.0508)
  line L556 (-50.0217, 52.5769) -> (-52.7477, 49.8508)
  line L557 (-52.7477, 49.8508) -> (-50.0748, 47.1779)
  line L558 (-50.0748, 47.1779) -> (-47.3488, 49.9039)
  line L559 (-47.3488, 49.9039) -> (-50.0217, 52.5769)
  line L560 (-50.0217, 52.5769) -> (-50.0748, 47.1779) construction
  line L561 (-52.7477, 49.8508) -> (-47.3488, 49.9039) construction
  line L562 (-38.0237, 52.5769) -> (-35.2976, 49.8508)
  line L563 (-35.2976, 49.8508) -> (-37.9706, 47.1779)
  line L564 (-37.9706, 47.1779) -> (-40.6966, 49.9039)
  line L565 (-40.6966, 49.9039) -> (-38.0237, 52.5769)
  line L566 (-14.2237, 52.5769) -> (-11.4976, 49.8508)
  line L567 (-11.4976, 49.8508) -> (-14.1706, 47.1779)
  line L568 (-14.1706, 47.1779) -> (-16.8966, 49.9039)
  line L569 (-16.8966, 49.9039) -> (-14.2237, 52.5769)
  line L570 (-23.5488, 49.9039) -> (-26.2217, 52.5769)
  line L571 (-26.2748, 47.1779) -> (-23.5488, 49.9039)
  line L572 (-28.9477, 49.8508) -> (-26.2748, 47.1779)
  line L573 (-26.2217, 52.5769) -> (-28.9477, 49.8508)
  line L574 (-50.0748, 41.1431) -> (-47.3488, 38.4171)
  line L575 (-47.3488, 38.4171) -> (-50.0217, 35.7442)
  line L576 (-50.0217, 35.7442) -> (-50.0748, 41.1431) construction
  line L577 (-52.7477, 38.4702) -> (-47.3488, 38.4171) construction
  line L578 (-50.0217, 35.7442) -> (-52.7477, 38.4702)
  line L579 (-52.7477, 38.4702) -> (-50.0748, 41.1431)
  line L580 (-40.6966, 38.4171) -> (-38.0237, 35.7442)
  line L581 (-37.9706, 41.1431) -> (-40.6966, 38.4171)
  line L582 (-38.0237, 35.7442) -> (-35.2976, 38.4702)
  line L583 (-35.2976, 38.4702) -> (-37.9706, 41.1431)
  line L584 (-26.2748, 41.1431) -> (-23.5488, 38.4171)
  line L585 (-23.5488, 38.4171) -> (-26.2217, 35.7442)
  line L586 (-28.9477, 38.4702) -> (-26.2748, 41.1431)
  line L587 (-26.2217, 35.7442) -> (-28.9477, 38.4702)
  line L588 (-14.1706, 41.1431) -> (-16.8966, 38.4171)
  line L589 (-11.4976, 38.4702) -> (-14.1706, 41.1431)
  line L590 (-16.8966, 38.4171) -> (-14.2237, 35.7442)
  line L591 (-14.2237, 35.7442) -> (-11.4976, 38.4702)
  line L592 (-50.0217, 100.1769) -> (-52.7477, 97.4508)
  line L593 (-52.7477, 97.4508) -> (-50.0748, 94.7779)
  line L594 (-50.0748, 94.7779) -> (-47.3488, 97.5039)
  line L595 (-47.3488, 97.5039) -> (-50.0217, 100.1769)
  line L596 (-50.0217, 100.1769) -> (-50.0748, 94.7779) construction
  line L597 (-52.7477, 97.4508) -> (-47.3488, 97.5039) construction
  line L598 (-38.0237, 100.1769) -> (-35.2976, 97.4508)
  line L599 (-35.2976, 97.4508) -> (-37.9706, 94.7779)
  line L600 (-37.9706, 94.7779) -> (-40.6966, 97.5039)
  line L601 (-40.6966, 97.5039) -> (-38.0237, 100.1769)
  line L602 (-14.2237, 100.1769) -> (-11.4976, 97.4508)
  line L603 (-11.4976, 97.4508) -> (-14.1706, 94.7779)
  line L604 (-14.1706, 94.7779) -> (-16.8966, 97.5039)
  line L605 (-16.8966, 97.5039) -> (-14.2237, 100.1769)
  line L606 (-23.5488, 97.5039) -> (-26.2217, 100.1769)
  line L607 (-26.2748, 94.7779) -> (-23.5488, 97.5039)
  line L608 (-28.9477, 97.4508) -> (-26.2748, 94.7779)
  line L609 (-26.2217, 100.1769) -> (-28.9477, 97.4508)
  line L610 (-50.0748, 88.7431) -> (-47.3488, 86.0171)
  line L611 (-47.3488, 86.0171) -> (-50.0217, 83.3442)
  line L612 (-50.0217, 83.3442) -> (-50.0748, 88.7431) construction
  line L613 (-52.7477, 86.0702) -> (-47.3488, 86.0171) construction
  line L614 (-50.0217, 83.3442) -> (-52.7477, 86.0702)
  line L615 (-52.7477, 86.0702) -> (-50.0748, 88.7431)
  line L616 (-40.6966, 86.0171) -> (-38.0237, 83.3442)
  line L617 (-37.9706, 88.7431) -> (-40.6966, 86.0171)
  line L618 (-38.0237, 83.3442) -> (-35.2976, 86.0702)
  line L619 (-35.2976, 86.0702) -> (-37.9706, 88.7431)
  line L620 (-26.2748, 88.7431) -> (-23.5488, 86.0171)
  line L621 (-23.5488, 86.0171) -> (-26.2217, 83.3442)
  line L622 (-28.9477, 86.0702) -> (-26.2748, 88.7431)
  line L623 (-26.2217, 83.3442) -> (-28.9477, 86.0702)
  line L624 (-14.1706, 88.7431) -> (-16.8966, 86.0171)
  line L625 (-11.4976, 86.0702) -> (-14.1706, 88.7431)
  line L626 (-16.8966, 86.0171) -> (-14.2237, 83.3442)
  line L627 (-14.2237, 83.3442) -> (-11.4976, 86.0702)
  line L628 (-50.0748, 70.9779) -> (-47.3488, 73.7039)
  line L629 (-50.0217, 76.3769) -> (-50.0748, 70.9779) construction
  line L630 (-52.7477, 73.6508) -> (-50.0748, 70.9779)
  line L631 (-52.7477, 73.6508) -> (-47.3488, 73.7039) construction
  line L632 (-50.0217, 76.3769) -> (-52.7477, 73.6508)
  line L633 (-47.3488, 73.7039) -> (-50.0217, 76.3769)
  line L634 (-50.0748, 64.9431) -> (-47.3488, 62.2171)
  line L635 (-47.3488, 62.2171) -> (-50.0217, 59.5442)
  line L636 (-50.0217, 59.5442) -> (-50.0748, 64.9431) construction
  line L637 (-52.7477, 62.2702) -> (-47.3488, 62.2171) construction
  line L638 (-52.7477, 62.2702) -> (-50.0748, 64.9431)
  line L639 (-50.0217, 59.5442) -> (-52.7477, 62.2702)
  line L640 (-40.6966, 73.7039) -> (-38.0237, 76.3769)
  line L641 (-37.9706, 70.9779) -> (-40.6966, 73.7039)
  line L642 (-38.0237, 76.3769) -> (-35.2976, 73.6508)
  line L643 (-35.2976, 73.6508) -> (-37.9706, 70.9779)
  line L644 (-35.2976, 62.2702) -> (-37.9706, 64.9431)
  line L645 (-37.9706, 64.9431) -> (-40.6966, 62.2171)
  line L646 (-38.0237, 59.5442) -> (-35.2976, 62.2702)
  line L647 (-40.6966, 62.2171) -> (-38.0237, 59.5442)
  line L648 (-28.9477, 62.2702) -> (-26.2748, 64.9431)
  line L649 (-26.2217, 59.5442) -> (-28.9477, 62.2702)
  line L650 (-23.5488, 62.2171) -> (-26.2217, 59.5442)
  line L651 (-26.2748, 64.9431) -> (-23.5488, 62.2171)
  line L652 (-28.9477, 73.6508) -> (-26.2748, 70.9779)
  line L653 (-26.2748, 70.9779) -> (-23.5488, 73.7039)
  line L654 (-26.2217, 76.3769) -> (-28.9477, 73.6508)
  line L655 (-23.5488, 73.7039) -> (-26.2217, 76.3769)
  line L656 (-14.2237, 59.5442) -> (-11.4976, 62.2702)
  line L657 (-16.8966, 62.2171) -> (-14.2237, 59.5442)
  line L658 (-11.4976, 62.2702) -> (-14.1706, 64.9431)
  line L659 (-14.1706, 64.9431) -> (-16.8966, 62.2171)
  line L660 (-11.4976, 73.6508) -> (-14.1706, 70.9779)
  line L661 (-14.1706, 70.9779) -> (-16.8966, 73.7039)
  line L662 (-14.2237, 76.3769) -> (-11.4976, 73.6508)
  line L663 (-16.8966, 73.7039) -> (-14.2237, 76.3769)
  line L664 (-50.0217, 195.3769) -> (-52.7477, 192.6508)
  line L665 (-52.7477, 192.6508) -> (-50.0748, 189.9779)
  line L666 (-50.0748, 189.9779) -> (-47.3488, 192.7039)
  line L667 (-47.3488, 192.7039) -> (-50.0217, 195.3769)
  line L668 (-50.0217, 195.3769) -> (-50.0748, 189.9779) construction
  line L669 (-52.7477, 192.6508) -> (-47.3488, 192.7039) construction
  line L670 (-38.0237, 195.3769) -> (-35.2976, 192.6508)
  line L671 (-35.2976, 192.6508) -> (-37.9706, 189.9779)
  line L672 (-37.9706, 189.9779) -> (-40.6966, 192.7039)
  line L673 (-40.6966, 192.7039) -> (-38.0237, 195.3769)
  line L674 (-14.2237, 195.3769) -> (-11.4976, 192.6508)
  line L675 (-11.4976, 192.6508) -> (-14.1706, 189.9779)
  line L676 (-14.1706, 189.9779) -> (-16.8966, 192.7039)
  line L677 (-16.8966, 192.7039) -> (-14.2237, 195.3769)
  line L678 (-23.5488, 192.7039) -> (-26.2217, 195.3769)
  line L679 (-26.2748, 189.9779) -> (-23.5488, 192.7039)
  line L680 (-28.9477, 192.6508) -> (-26.2748, 189.9779)
  line L681 (-26.2217, 195.3769) -> (-28.9477, 192.6508)
  line L682 (-50.0748, 183.9431) -> (-47.3488, 181.2171)
  line L683 (-47.3488, 181.2171) -> (-50.0217, 178.5442)
  line L684 (-50.0217, 178.5442) -> (-50.0748, 183.9431) construction
  line L685 (-52.7477, 181.2702) -> (-47.3488, 181.2171) construction
  line L686 (-50.0217, 178.5442) -> (-52.7477, 181.2702)
  line L687 (-52.7477, 181.2702) -> (-50.0748, 183.9431)
  line L688 (-40.6966, 181.2171) -> (-38.0237, 178.5442)
  line L689 (-37.9706, 183.9431) -> (-40.6966, 181.2171)
  line L690 (-38.0237, 178.5442) -> (-35.2976, 181.2702)
  line L691 (-35.2976, 181.2702) -> (-37.9706, 183.9431)
  line L692 (-26.2748, 183.9431) -> (-23.5488, 181.2171)
  line L693 (-23.5488, 181.2171) -> (-26.2217, 178.5442)
  line L694 (-28.9477, 181.2702) -> (-26.2748, 183.9431)
  line L695 (-26.2217, 178.5442) -> (-28.9477, 181.2702)
  line L696 (-14.1706, 183.9431) -> (-16.8966, 181.2171)
  line L697 (-11.4976, 181.2702) -> (-14.1706, 183.9431)
  line L698 (-16.8966, 181.2171) -> (-14.2237, 178.5442)
  line L699 (-14.2237, 178.5442) -> (-11.4976, 181.2702)
  line L700 (-50.0748, 166.1779) -> (-47.3488, 168.9039)
  line L701 (-50.0217, 171.5769) -> (-50.0748, 166.1779) construction
  line L702 (-52.7477, 168.8508) -> (-50.0748, 166.1779)
  line L703 (-52.7477, 168.8508) -> (-47.3488, 168.9039) construction
  line L704 (-50.0217, 171.5769) -> (-52.7477, 168.8508)
  line L705 (-47.3488, 168.9039) -> (-50.0217, 171.5769)
  line L706 (-50.0748, 160.1431) -> (-47.3488, 157.4171)
  line L707 (-47.3488, 157.4171) -> (-50.0217, 154.7442)
  line L708 (-50.0217, 154.7442) -> (-50.0748, 160.1431) construction
  line L709 (-52.7477, 157.4702) -> (-47.3488, 157.4171) construction
  line L710 (-52.7477, 157.4702) -> (-50.0748, 160.1431)
  line L711 (-50.0217, 154.7442) -> (-52.7477, 157.4702)
  line L712 (-40.6966, 168.9039) -> (-38.0237, 171.5769)
  line L713 (-37.9706, 166.1779) -> (-40.6966, 168.9039)
  line L714 (-38.0237, 171.5769) -> (-35.2976, 168.8508)
  line L715 (-35.2976, 168.8508) -> (-37.9706, 166.1779)
  line L716 (-35.2976, 157.4702) -> (-37.9706, 160.1431)
  line L717 (-37.9706, 160.1431) -> (-40.6966, 157.4171)
  line L718 (-38.0237, 154.7442) -> (-35.2976, 157.4702)
  line L719 (-40.6966, 157.4171) -> (-38.0237, 154.7442)
  line L720 (-28.9477, 157.4702) -> (-26.2748, 160.1431)
  line L721 (-26.2217, 154.7442) -> (-28.9477, 157.4702)
  line L722 (-23.5488, 157.4171) -> (-26.2217, 154.7442)
  line L723 (-26.2748, 160.1431) -> (-23.5488, 157.4171)
  line L724 (-28.9477, 168.8508) -> (-26.2748, 166.1779)
  line L725 (-26.2748, 166.1779) -> (-23.5488, 168.9039)
  line L726 (-26.2217, 171.5769) -> (-28.9477, 168.8508)
  line L727 (-23.5488, 168.9039) -> (-26.2217, 171.5769)
  line L728 (-14.2237, 154.7442) -> (-11.4976, 157.4702)
  line L729 (-16.8966, 157.4171) -> (-14.2237, 154.7442)
  line L730 (-11.4976, 157.4702) -> (-14.1706, 160.1431)
  line L731 (-14.1706, 160.1431) -> (-16.8966, 157.4171)
  line L732 (-11.4976, 168.8508) -> (-14.1706, 166.1779)
  line L733 (-14.1706, 166.1779) -> (-16.8966, 168.9039)
  line L734 (-14.2237, 171.5769) -> (-11.4976, 168.8508)
  line L735 (-16.8966, 168.9039) -> (-14.2237, 171.5769)
  line L736 (-52.7477, 109.8702) -> (-50.0748, 112.5431)
  line L737 (-50.0748, 112.5431) -> (-47.3488, 109.8171)
  line L738 (-52.7477, 109.8702) -> (-47.3488, 109.8171) construction
  line L739 (-47.3488, 109.8171) -> (-50.0217, 107.1442)
  line L740 (-50.0217, 107.1442) -> (-52.7477, 109.8702)
  line L741 (-50.0217, 107.1442) -> (-50.0748, 112.5431) construction
  line L742 (-50.0217, 147.7769) -> (-50.0748, 142.3779) construction
  line L743 (-50.0748, 142.3779) -> (-47.3488, 145.1039)
  line L744 (-47.3488, 145.1039) -> (-50.0217, 147.7769)
  line L745 (-52.7477, 145.0508) -> (-47.3488, 145.1039) construction
  line L746 (-50.0217, 147.7769) -> (-52.7477, 145.0508)
  line L747 (-50.0217, 130.9442) -> (-52.7477, 133.6702)
  line L748 (-52.7477, 133.6702) -> (-47.3488, 133.6171) construction
  line L749 (-52.7477, 133.6702) -> (-50.0748, 136.3431)
  line L750 (-47.3488, 133.6171) -> (-50.0217, 130.9442)
  line L751 (-50.0217, 130.9442) -> (-50.0748, 136.3431) construction
  line L752 (-50.0748, 136.3431) -> (-47.3488, 133.6171)
  line L753 (-52.7477, 121.2508) -> (-50.0748, 118.5779)
  line L754 (-50.0748, 118.5779) -> (-47.3488, 121.3039)
  line L755 (-50.0217, 123.9769) -> (-50.0748, 118.5779) construction
  line L756 (-50.0217, 123.9769) -> (-52.7477, 121.2508)
  line L757 (-47.3488, 121.3039) -> (-50.0217, 123.9769)
  line L758 (-52.7477, 121.2508) -> (-47.3488, 121.3039) construction
  line L759 (-52.7477, 145.0508) -> (-50.0748, 142.3779)
  line L760 (-35.2976, 145.0508) -> (-37.9706, 142.3779)
  line L761 (-38.0237, 147.7769) -> (-35.2976, 145.0508)
  line L762 (-37.9706, 142.3779) -> (-40.6966, 145.1039)
  line L763 (-40.6966, 145.1039) -> (-38.0237, 147.7769)
  line L764 (-40.6966, 133.6171) -> (-38.0237, 130.9442)
  line L765 (-37.9706, 136.3431) -> (-40.6966, 133.6171)
  line L766 (-38.0237, 130.9442) -> (-35.2976, 133.6702)
  line L767 (-35.2976, 133.6702) -> (-37.9706, 136.3431)
  line L768 (-40.6966, 109.8171) -> (-38.0237, 107.1442)
  line L769 (-37.9706, 112.5431) -> (-40.6966, 109.8171)
  line L770 (-38.0237, 107.1442) -> (-35.2976, 109.8702)
  line L771 (-35.2976, 109.8702) -> (-37.9706, 112.5431)
  line L772 (-37.9706, 118.5779) -> (-40.6966, 121.3039)
  line L773 (-35.2976, 121.2508) -> (-37.9706, 118.5779)
  line L774 (-40.6966, 121.3039) -> (-38.0237, 123.9769)
  line L775 (-38.0237, 123.9769) -> (-35.2976, 121.2508)
  line L776 (-28.9477, 145.0508) -> (-26.2748, 142.3779)
  line L777 (-26.2217, 147.7769) -> (-28.9477, 145.0508)
  line L778 (-26.2748, 142.3779) -> (-23.5488, 145.1039)
  line L779 (-23.5488, 145.1039) -> (-26.2217, 147.7769)
  line L780 (-23.5488, 133.6171) -> (-26.2217, 130.9442)
  line L781 (-26.2217, 130.9442) -> (-28.9477, 133.6702)
  line L782 (-28.9477, 133.6702) -> (-26.2748, 136.3431)
  line L783 (-26.2748, 136.3431) -> (-23.5488, 133.6171)
  line L784 (-26.2217, 123.9769) -> (-28.9477, 121.2508)
  line L785 (-23.5488, 109.8171) -> (-26.2217, 107.1442)
  line L786 (-26.2748, 112.5431) -> (-23.5488, 109.8171)
  line L787 (-26.2217, 107.1442) -> (-28.9477, 109.8702)
  line L788 (-28.9477, 109.8702) -> (-26.2748, 112.5431)
  line L789 (-26.2748, 118.5779) -> (-23.5488, 121.3039)
  line L790 (-23.5488, 121.3039) -> (-26.2217, 123.9769)
  line L791 (-28.9477, 121.2508) -> (-26.2748, 118.5779)
  line L792 (-16.8966, 145.1039) -> (-14.2237, 147.7769)
  line L793 (-14.1706, 142.3779) -> (-16.8966, 145.1039)
  line L794 (-11.4976, 145.0508) -> (-14.1706, 142.3779)
  line L795 (-14.2237, 147.7769) -> (-11.4976, 145.0508)
  line L796 (-16.8966, 133.6171) -> (-14.2237, 130.9442)
  line L797 (-14.1706, 136.3431) -> (-16.8966, 133.6171)
  line L798 (-11.4976, 133.6702) -> (-14.1706, 136.3431)
  line L799 (-14.2237, 130.9442) -> (-11.4976, 133.6702)
  line L800 (-16.8966, 109.8171) -> (-14.2237, 107.1442)
  line L801 (-11.4976, 109.8702) -> (-14.1706, 112.5431)
  line L802 (-14.2237, 107.1442) -> (-11.4976, 109.8702)
  line L803 (-14.1706, 112.5431) -> (-16.8966, 109.8171)
  line L804 (-14.1706, 118.5779) -> (-16.8966, 121.3039)
  line L805 (-11.4976, 121.2508) -> (-14.1706, 118.5779)
  line L806 (-16.8966, 121.3039) -> (-14.2237, 123.9769)
  line L807 (-14.2237, 123.9769) -> (-11.4976, 121.2508)
  line L808 (-58.2087, 198.8605) -> (-6.0367, 198.8605)
  line L809 (-10.6087, 201.1465) -> (-6.0367, 201.1465)
  line L810 (-52.7477, 300.2702) -> (-50.0748, 302.9431)
  line L811 (-50.0748, 302.9431) -> (-47.3488, 300.2171)
  line L812 (-52.7477, 300.2702) -> (-47.3488, 300.2171) construction
  line L813 (-47.3488, 300.2171) -> (-50.0217, 297.5442)
  line L814 (-50.0217, 297.5442) -> (-52.7477, 300.2702)
  line L815 (-50.0217, 297.5442) -> (-50.0748, 302.9431) construction
  line L816 (-40.6966, 300.2171) -> (-38.0237, 297.5442)
  line L817 (-37.9706, 302.9431) -> (-40.6966, 300.2171)
  line L818 (-38.0237, 297.5442) -> (-35.2976, 300.2702)
  line L819 (-35.2976, 300.2702) -> (-37.9706, 302.9431)
  line L820 (-23.5488, 300.2171) -> (-26.2217, 297.5442)
  line L821 (-26.2748, 302.9431) -> (-23.5488, 300.2171)
  line L822 (-26.2217, 297.5442) -> (-28.9477, 300.2702)
  line L823 (-28.9477, 300.2702) -> (-26.2748, 302.9431)
  line L824 (-16.8966, 300.2171) -> (-14.2237, 297.5442)
  line L825 (-11.4976, 300.2702) -> (-14.1706, 302.9431)
  line L826 (-14.2237, 297.5442) -> (-11.4976, 300.2702)
  line L827 (-14.1706, 302.9431) -> (-16.8966, 300.2171)
  line L828 (-50.0748, 261.3779) -> (-47.3488, 264.1039)
  line L829 (-52.7477, 264.0508) -> (-50.0748, 261.3779)
  line L830 (-52.7477, 264.0508) -> (-47.3488, 264.1039) construction
  line L831 (-50.0217, 266.7769) -> (-50.0748, 261.3779) construction
  line L832 (-47.3488, 264.1039) -> (-50.0217, 266.7769)
  line L833 (-50.0217, 266.7769) -> (-52.7477, 264.0508)
  line L834 (-52.7477, 276.4702) -> (-50.0748, 279.1431)
  line L835 (-50.0748, 279.1431) -> (-47.3488, 276.4171)
  line L836 (-52.7477, 276.4702) -> (-47.3488, 276.4171) construction
  line L837 (-50.0217, 273.7442) -> (-50.0748, 279.1431) construction
  line L838 (-50.0217, 273.7442) -> (-52.7477, 276.4702)
  line L839 (-47.3488, 276.4171) -> (-50.0217, 273.7442)
  line L840 (-52.7477, 287.8508) -> (-50.0748, 285.1779)
  line L841 (-50.0748, 285.1779) -> (-47.3488, 287.9039)
  line L842 (-52.7477, 287.8508) -> (-47.3488, 287.9039) construction
  line L843 (-50.0217, 290.5769) -> (-50.0748, 285.1779) construction
  line L844 (-50.0217, 290.5769) -> (-52.7477, 287.8508)
  line L845 (-47.3488, 287.9039) -> (-50.0217, 290.5769)
  line L846 (-52.7477, 252.6702) -> (-50.0748, 255.3431)
  line L847 (-52.7477, 252.6702) -> (-47.3488, 252.6171) construction
  line L848 (-50.0217, 249.9442) -> (-52.7477, 252.6702)
  line L849 (-50.0217, 249.9442) -> (-50.0748, 255.3431) construction
  line L850 (-47.3488, 252.6171) -> (-50.0217, 249.9442)
  line L851 (-50.0748, 255.3431) -> (-47.3488, 252.6171)
  line L852 (-52.7477, 240.2508) -> (-50.0748, 237.5779)
  line L853 (-50.0217, 242.9769) -> (-52.7477, 240.2508)
  line L854 (-52.7477, 240.2508) -> (-47.3488, 240.3039) construction
  line L855 (-50.0217, 242.9769) -> (-50.0748, 237.5779) construction
  line L856 (-50.0748, 237.5779) -> (-47.3488, 240.3039)
  line L857 (-47.3488, 240.3039) -> (-50.0217, 242.9769)
  line L858 (-52.7477, 216.4508) -> (-50.0748, 213.7779)
  line L859 (-50.0217, 219.1769) -> (-52.7477, 216.4508)
  line L860 (-50.0748, 213.7779) -> (-47.3488, 216.5039)
  line L861 (-52.7477, 216.4508) -> (-47.3488, 216.5039) construction